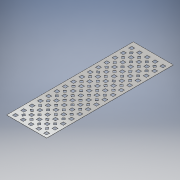
# Autodesk Inventor part: flat metal frame
Saved by Autodesk Inventor 2018 (Build 220112000, 112)
## iProperties
Created: 2018-10-16
Part Number: flat metal frame
Material: Generic
Document SubType Name: Modeling
Designer: USER
Density: 1 g/cm^3
Appearance: Machined - Aluminum
Author: USER
Autodesk Inventor part; units mm, degrees
ref_plane "YZ Plane" through (0, 0, 0) normal (1, 0, 0) x (0, 1, 0)
ref_plane "XZ Plane" through (0, 0, 0) normal (0, 1, 0) x (-1, 0, 0)
ref_plane "XY Plane" through (0, 0, 0) normal (0, 0, 1) x (1, 0, 0)
sketch "Sketch1" plane through (0, 0, 0) normal (0, 1, 0) x (-1, 0, 0)
  line L0 (0, 0) -> (59.9948, 0)
  line L1 (59.9948, 0) -> (59.9948, -189.992)
  line L2 (59.9948, -189.992) -> (0, -189.992)
  line L3 (0, -189.992) -> (0, 0)
  dimension "d0" = 59.9948
  dimension "d1" = 189.992
  constraints: 8 end point, 2 parallel, 1 horizontal, 1 perpendicular
  measures "d0" distance of L1.end L2.end
  measures "d1" distance of L0.end L1.end
extrude "Extrusion1" add sketch "Sketch1" against normal blind 0.254
sketch "Sketch2" plane through (0, 0, 0) normal (0, 1, 0) x (1, 0, 0)
  line L0 (-4.0386, 4.0386) -> (-8.6106, 4.0386)
  line L1 (-8.6106, 4.0386) -> (-8.6106, 8.6106)
  line L2 (-8.6106, 8.6106) -> (-4.0386, 8.6106)
  line L3 (-4.0386, 8.6106) -> (-4.0386, 4.0386)
  line L4 (-15.7226, 4.0386) -> (-20.2946, 4.0386)
  line L5 (-20.2946, 4.0386) -> (-20.2946, 8.6106)
  line L6 (-20.2946, 8.6106) -> (-15.7226, 8.6106)
  line L7 (-15.7226, 8.6106) -> (-15.7226, 4.0386)
  line L8 (-27.4066, 4.0386) -> (-31.9786, 4.0386)
  line L9 (-31.9786, 4.0386) -> (-31.9786, 8.6106)
  line L10 (-31.9786, 8.6106) -> (-27.4066, 8.6106)
  line L11 (-27.4066, 8.6106) -> (-27.4066, 4.0386)
  line L12 (-39.0906, 4.0386) -> (-43.6626, 4.0386)
  line L13 (-43.6626, 4.0386) -> (-43.6626, 8.6106)
  line L14 (-43.6626, 8.6106) -> (-39.0906, 8.6106)
  line L15 (-39.0906, 8.6106) -> (-39.0906, 4.0386)
  line L16 (-50.7746, 4.0386) -> (-55.3466, 4.0386)
  line L17 (-55.3466, 4.0386) -> (-55.3466, 8.6106)
  line L18 (-55.3466, 8.6106) -> (-50.7746, 8.6106)
  line L19 (-50.7746, 8.6106) -> (-50.7746, 4.0386)
  line L20 (-39.0906, 21.0566) -> (-39.0906, 16.4846)
  line L21 (-39.0906, 16.4846) -> (-43.6626, 16.4846)
  line L22 (-43.6626, 21.0566) -> (-39.0906, 21.0566)
  line L23 (-43.6626, 16.4846) -> (-43.6626, 21.0566)
  line L24 (-50.7746, 21.0566) -> (-50.7746, 16.4846)
  line L25 (-55.3466, 21.0566) -> (-50.7746, 21.0566)
  line L26 (-4.0386, 16.4846) -> (-8.6106, 16.4846)
  line L27 (-8.6106, 16.4846) -> (-8.6106, 21.0566)
  line L28 (-8.6106, 21.0566) -> (-4.0386, 21.0566)
  line L29 (-31.9786, 16.4846) -> (-31.9786, 21.0566)
  line L30 (-27.4066, 16.4846) -> (-31.9786, 16.4846)
  line L31 (-27.4066, 21.0566) -> (-27.4066, 16.4846)
  line L32 (-20.2946, 16.4846) -> (-20.2946, 21.0566)
  line L33 (-15.7226, 16.4846) -> (-20.2946, 16.4846)
  line L34 (-20.2946, 21.0566) -> (-15.7226, 21.0566)
  line L35 (-15.7226, 21.0566) -> (-15.7226, 16.4846)
  line L36 (-4.0386, 21.0566) -> (-4.0386, 16.4846)
  line L37 (-31.9786, 21.0566) -> (-27.4066, 21.0566)
  line L38 (-55.3466, 16.4846) -> (-55.3466, 21.0566)
  line L39 (-50.7746, 16.4846) -> (-55.3466, 16.4846)
  line L40 (-39.0906, 33.5026) -> (-39.0906, 28.9306)
  line L41 (-39.0906, 28.9306) -> (-43.6626, 28.9306)
  line L42 (-43.6626, 33.5026) -> (-39.0906, 33.5026)
  line L43 (-43.6626, 28.9306) -> (-43.6626, 33.5026)
  line L44 (-50.7746, 33.5026) -> (-50.7746, 28.9306)
  line L45 (-55.3466, 33.5026) -> (-50.7746, 33.5026)
  line L46 (-4.0386, 28.9306) -> (-8.6106, 28.9306)
  line L47 (-8.6106, 28.9306) -> (-8.6106, 33.5026)
  line L48 (-8.6106, 33.5026) -> (-4.0386, 33.5026)
  line L49 (-31.9786, 28.9306) -> (-31.9786, 33.5026)
  line L50 (-27.4066, 28.9306) -> (-31.9786, 28.9306)
  line L51 (-27.4066, 33.5026) -> (-27.4066, 28.9306)
  line L52 (-20.2946, 28.9306) -> (-20.2946, 33.5026)
  line L53 (-15.7226, 28.9306) -> (-20.2946, 28.9306)
  line L54 (-20.2946, 33.5026) -> (-15.7226, 33.5026)
  line L55 (-15.7226, 33.5026) -> (-15.7226, 28.9306)
  line L56 (-4.0386, 33.5026) -> (-4.0386, 28.9306)
  line L57 (-31.9786, 33.5026) -> (-27.4066, 33.5026)
  line L58 (-55.3466, 28.9306) -> (-55.3466, 33.5026)
  line L59 (-50.7746, 28.9306) -> (-55.3466, 28.9306)
  line L60 (-39.0906, 45.9486) -> (-39.0906, 41.3766)
  line L61 (-39.0906, 41.3766) -> (-43.6626, 41.3766)
  line L62 (-43.6626, 45.9486) -> (-39.0906, 45.9486)
  line L63 (-43.6626, 41.3766) -> (-43.6626, 45.9486)
  line L64 (-50.7746, 45.9486) -> (-50.7746, 41.3766)
  line L65 (-55.3466, 45.9486) -> (-50.7746, 45.9486)
  line L66 (-4.0386, 41.3766) -> (-8.6106, 41.3766)
  line L67 (-8.6106, 41.3766) -> (-8.6106, 45.9486)
  line L68 (-8.6106, 45.9486) -> (-4.0386, 45.9486)
  line L69 (-31.9786, 41.3766) -> (-31.9786, 45.9486)
  line L70 (-27.4066, 41.3766) -> (-31.9786, 41.3766)
  line L71 (-27.4066, 45.9486) -> (-27.4066, 41.3766)
  line L72 (-20.2946, 41.3766) -> (-20.2946, 45.9486)
  line L73 (-15.7226, 41.3766) -> (-20.2946, 41.3766)
  line L74 (-20.2946, 45.9486) -> (-15.7226, 45.9486)
  line L75 (-15.7226, 45.9486) -> (-15.7226, 41.3766)
  line L76 (-4.0386, 45.9486) -> (-4.0386, 41.3766)
  line L77 (-31.9786, 45.9486) -> (-27.4066, 45.9486)
  line L78 (-55.3466, 41.3766) -> (-55.3466, 45.9486)
  line L79 (-50.7746, 41.3766) -> (-55.3466, 41.3766)
  line L80 (-39.0906, 58.3946) -> (-39.0906, 53.8226)
  line L81 (-39.0906, 53.8226) -> (-43.6626, 53.8226)
  line L82 (-43.6626, 58.3946) -> (-39.0906, 58.3946)
  line L83 (-43.6626, 53.8226) -> (-43.6626, 58.3946)
  line L84 (-50.7746, 58.3946) -> (-50.7746, 53.8226)
  line L85 (-55.3466, 58.3946) -> (-50.7746, 58.3946)
  line L86 (-4.0386, 53.8226) -> (-8.6106, 53.8226)
  line L87 (-8.6106, 53.8226) -> (-8.6106, 58.3946)
  line L88 (-8.6106, 58.3946) -> (-4.0386, 58.3946)
  line L89 (-31.9786, 53.8226) -> (-31.9786, 58.3946)
  line L90 (-27.4066, 53.8226) -> (-31.9786, 53.8226)
  line L91 (-27.4066, 58.3946) -> (-27.4066, 53.8226)
  line L92 (-20.2946, 53.8226) -> (-20.2946, 58.3946)
  line L93 (-15.7226, 53.8226) -> (-20.2946, 53.8226)
  line L94 (-20.2946, 58.3946) -> (-15.7226, 58.3946)
  line L95 (-15.7226, 58.3946) -> (-15.7226, 53.8226)
  line L96 (-4.0386, 58.3946) -> (-4.0386, 53.8226)
  line L97 (-31.9786, 58.3946) -> (-27.4066, 58.3946)
  line L98 (-55.3466, 53.8226) -> (-55.3466, 58.3946)
  line L99 (-50.7746, 53.8226) -> (-55.3466, 53.8226)
  line L100 (-39.0906, 70.8406) -> (-39.0906, 66.2686)
  line L101 (-39.0906, 66.2686) -> (-43.6626, 66.2686)
  line L102 (-43.6626, 70.8406) -> (-39.0906, 70.8406)
  line L103 (-43.6626, 66.2686) -> (-43.6626, 70.8406)
  line L104 (-50.7746, 70.8406) -> (-50.7746, 66.2686)
  line L105 (-55.3466, 70.8406) -> (-50.7746, 70.8406)
  line L106 (-4.0386, 66.2686) -> (-8.6106, 66.2686)
  line L107 (-8.6106, 66.2686) -> (-8.6106, 70.8406)
  line L108 (-8.6106, 70.8406) -> (-4.0386, 70.8406)
  line L109 (-31.9786, 66.2686) -> (-31.9786, 70.8406)
  line L110 (-27.4066, 66.2686) -> (-31.9786, 66.2686)
  line L111 (-27.4066, 70.8406) -> (-27.4066, 66.2686)
  line L112 (-20.2946, 66.2686) -> (-20.2946, 70.8406)
  line L113 (-15.7226, 66.2686) -> (-20.2946, 66.2686)
  line L114 (-20.2946, 70.8406) -> (-15.7226, 70.8406)
  line L115 (-15.7226, 70.8406) -> (-15.7226, 66.2686)
  line L116 (-4.0386, 70.8406) -> (-4.0386, 66.2686)
  line L117 (-31.9786, 70.8406) -> (-27.4066, 70.8406)
  line L118 (-55.3466, 66.2686) -> (-55.3466, 70.8406)
  line L119 (-50.7746, 66.2686) -> (-55.3466, 66.2686)
  line L120 (-39.0906, 83.2866) -> (-39.0906, 78.7146)
  line L121 (-39.0906, 78.7146) -> (-43.6626, 78.7146)
  line L122 (-43.6626, 83.2866) -> (-39.0906, 83.2866)
  line L123 (-43.6626, 78.7146) -> (-43.6626, 83.2866)
  line L124 (-50.7746, 83.2866) -> (-50.7746, 78.7146)
  line L125 (-55.3466, 83.2866) -> (-50.7746, 83.2866)
  line L126 (-4.0386, 78.7146) -> (-8.6106, 78.7146)
  line L127 (-8.6106, 78.7146) -> (-8.6106, 83.2866)
  line L128 (-8.6106, 83.2866) -> (-4.0386, 83.2866)
  line L129 (-31.9786, 78.7146) -> (-31.9786, 83.2866)
  line L130 (-27.4066, 78.7146) -> (-31.9786, 78.7146)
  line L131 (-27.4066, 83.2866) -> (-27.4066, 78.7146)
  line L132 (-20.2946, 78.7146) -> (-20.2946, 83.2866)
  line L133 (-15.7226, 78.7146) -> (-20.2946, 78.7146)
  line L134 (-20.2946, 83.2866) -> (-15.7226, 83.2866)
  line L135 (-15.7226, 83.2866) -> (-15.7226, 78.7146)
  line L136 (-4.0386, 83.2866) -> (-4.0386, 78.7146)
  line L137 (-31.9786, 83.2866) -> (-27.4066, 83.2866)
  line L138 (-55.3466, 78.7146) -> (-55.3466, 83.2866)
  line L139 (-50.7746, 78.7146) -> (-55.3466, 78.7146)
  line L140 (-39.0906, 95.7326) -> (-39.0906, 91.1606)
  line L141 (-39.0906, 91.1606) -> (-43.6626, 91.1606)
  line L142 (-43.6626, 95.7326) -> (-39.0906, 95.7326)
  line L143 (-43.6626, 91.1606) -> (-43.6626, 95.7326)
  line L144 (-50.7746, 95.7326) -> (-50.7746, 91.1606)
  line L145 (-55.3466, 95.7326) -> (-50.7746, 95.7326)
  line L146 (-4.0386, 91.1606) -> (-8.6106, 91.1606)
  line L147 (-8.6106, 91.1606) -> (-8.6106, 95.7326)
  line L148 (-8.6106, 95.7326) -> (-4.0386, 95.7326)
  line L149 (-31.9786, 91.1606) -> (-31.9786, 95.7326)
  line L150 (-27.4066, 91.1606) -> (-31.9786, 91.1606)
  line L151 (-27.4066, 95.7326) -> (-27.4066, 91.1606)
  line L152 (-20.2946, 91.1606) -> (-20.2946, 95.7326)
  line L153 (-15.7226, 91.1606) -> (-20.2946, 91.1606)
  line L154 (-20.2946, 95.7326) -> (-15.7226, 95.7326)
  line L155 (-15.7226, 95.7326) -> (-15.7226, 91.1606)
  line L156 (-4.0386, 95.7326) -> (-4.0386, 91.1606)
  line L157 (-31.9786, 95.7326) -> (-27.4066, 95.7326)
  line L158 (-55.3466, 91.1606) -> (-55.3466, 95.7326)
  line L159 (-50.7746, 91.1606) -> (-55.3466, 91.1606)
  line L160 (-39.0906, 108.1786) -> (-39.0906, 103.6066)
  line L161 (-39.0906, 103.6066) -> (-43.6626, 103.6066)
  line L162 (-43.6626, 108.1786) -> (-39.0906, 108.1786)
  line L163 (-43.6626, 103.6066) -> (-43.6626, 108.1786)
  line L164 (-50.7746, 108.1786) -> (-50.7746, 103.6066)
  line L165 (-55.3466, 108.1786) -> (-50.7746, 108.1786)
  line L166 (-4.0386, 103.6066) -> (-8.6106, 103.6066)
  line L167 (-8.6106, 103.6066) -> (-8.6106, 108.1786)
  line L168 (-8.6106, 108.1786) -> (-4.0386, 108.1786)
  line L169 (-31.9786, 103.6066) -> (-31.9786, 108.1786)
  line L170 (-27.4066, 103.6066) -> (-31.9786, 103.6066)
  line L171 (-27.4066, 108.1786) -> (-27.4066, 103.6066)
  line L172 (-20.2946, 103.6066) -> (-20.2946, 108.1786)
  line L173 (-15.7226, 103.6066) -> (-20.2946, 103.6066)
  line L174 (-20.2946, 108.1786) -> (-15.7226, 108.1786)
  line L175 (-15.7226, 108.1786) -> (-15.7226, 103.6066)
  line L176 (-4.0386, 108.1786) -> (-4.0386, 103.6066)
  line L177 (-31.9786, 108.1786) -> (-27.4066, 108.1786)
  line L178 (-55.3466, 103.6066) -> (-55.3466, 108.1786)
  line L179 (-50.7746, 103.6066) -> (-55.3466, 103.6066)
  line L180 (-39.0906, 120.6246) -> (-39.0906, 116.0526)
  line L181 (-39.0906, 116.0526) -> (-43.6626, 116.0526)
  line L182 (-43.6626, 120.6246) -> (-39.0906, 120.6246)
  line L183 (-43.6626, 116.0526) -> (-43.6626, 120.6246)
  line L184 (-50.7746, 120.6246) -> (-50.7746, 116.0526)
  line L185 (-55.3466, 120.6246) -> (-50.7746, 120.6246)
  line L186 (-4.0386, 116.0526) -> (-8.6106, 116.0526)
  line L187 (-8.6106, 116.0526) -> (-8.6106, 120.6246)
  line L188 (-8.6106, 120.6246) -> (-4.0386, 120.6246)
  line L189 (-31.9786, 116.0526) -> (-31.9786, 120.6246)
  line L190 (-27.4066, 116.0526) -> (-31.9786, 116.0526)
  line L191 (-27.4066, 120.6246) -> (-27.4066, 116.0526)
  line L192 (-20.2946, 116.0526) -> (-20.2946, 120.6246)
  line L193 (-15.7226, 116.0526) -> (-20.2946, 116.0526)
  line L194 (-20.2946, 120.6246) -> (-15.7226, 120.6246)
  line L195 (-15.7226, 120.6246) -> (-15.7226, 116.0526)
  line L196 (-4.0386, 120.6246) -> (-4.0386, 116.0526)
  line L197 (-31.9786, 120.6246) -> (-27.4066, 120.6246)
  line L198 (-55.3466, 116.0526) -> (-55.3466, 120.6246)
  line L199 (-50.7746, 116.0526) -> (-55.3466, 116.0526)
  line L200 (-39.0906, 133.0706) -> (-39.0906, 128.4986)
  line L201 (-39.0906, 128.4986) -> (-43.6626, 128.4986)
  line L202 (-43.6626, 133.0706) -> (-39.0906, 133.0706)
  line L203 (-43.6626, 128.4986) -> (-43.6626, 133.0706)
  line L204 (-50.7746, 133.0706) -> (-50.7746, 128.4986)
  line L205 (-55.3466, 133.0706) -> (-50.7746, 133.0706)
  line L206 (-4.0386, 128.4986) -> (-8.6106, 128.4986)
  line L207 (-8.6106, 128.4986) -> (-8.6106, 133.0706)
  line L208 (-8.6106, 133.0706) -> (-4.0386, 133.0706)
  line L209 (-31.9786, 128.4986) -> (-31.9786, 133.0706)
  line L210 (-27.4066, 128.4986) -> (-31.9786, 128.4986)
  line L211 (-27.4066, 133.0706) -> (-27.4066, 128.4986)
  line L212 (-20.2946, 128.4986) -> (-20.2946, 133.0706)
  line L213 (-15.7226, 128.4986) -> (-20.2946, 128.4986)
  line L214 (-20.2946, 133.0706) -> (-15.7226, 133.0706)
  line L215 (-15.7226, 133.0706) -> (-15.7226, 128.4986)
  line L216 (-4.0386, 133.0706) -> (-4.0386, 128.4986)
  line L217 (-31.9786, 133.0706) -> (-27.4066, 133.0706)
  line L218 (-55.3466, 128.4986) -> (-55.3466, 133.0706)
  line L219 (-50.7746, 128.4986) -> (-55.3466, 128.4986)
  line L220 (-39.0906, 145.5166) -> (-39.0906, 140.9446)
  line L221 (-39.0906, 140.9446) -> (-43.6626, 140.9446)
  line L222 (-43.6626, 145.5166) -> (-39.0906, 145.5166)
  line L223 (-43.6626, 140.9446) -> (-43.6626, 145.5166)
  line L224 (-50.7746, 145.5166) -> (-50.7746, 140.9446)
  line L225 (-55.3466, 145.5166) -> (-50.7746, 145.5166)
  line L226 (-4.0386, 140.9446) -> (-8.6106, 140.9446)
  line L227 (-8.6106, 140.9446) -> (-8.6106, 145.5166)
  line L228 (-8.6106, 145.5166) -> (-4.0386, 145.5166)
  line L229 (-31.9786, 140.9446) -> (-31.9786, 145.5166)
  line L230 (-27.4066, 140.9446) -> (-31.9786, 140.9446)
  line L231 (-27.4066, 145.5166) -> (-27.4066, 140.9446)
  line L232 (-20.2946, 140.9446) -> (-20.2946, 145.5166)
  line L233 (-15.7226, 140.9446) -> (-20.2946, 140.9446)
  line L234 (-20.2946, 145.5166) -> (-15.7226, 145.5166)
  line L235 (-15.7226, 145.5166) -> (-15.7226, 140.9446)
  line L236 (-4.0386, 145.5166) -> (-4.0386, 140.9446)
  line L237 (-31.9786, 145.5166) -> (-27.4066, 145.5166)
  line L238 (-55.3466, 140.9446) -> (-55.3466, 145.5166)
  line L239 (-50.7746, 140.9446) -> (-55.3466, 140.9446)
  line L240 (-39.0906, 157.9626) -> (-39.0906, 153.3906)
  line L241 (-39.0906, 153.3906) -> (-43.6626, 153.3906)
  line L242 (-43.6626, 157.9626) -> (-39.0906, 157.9626)
  line L243 (-43.6626, 153.3906) -> (-43.6626, 157.9626)
  line L244 (-50.7746, 157.9626) -> (-50.7746, 153.3906)
  line L245 (-55.3466, 157.9626) -> (-50.7746, 157.9626)
  line L246 (-4.0386, 153.3906) -> (-8.6106, 153.3906)
  line L247 (-8.6106, 153.3906) -> (-8.6106, 157.9626)
  line L248 (-8.6106, 157.9626) -> (-4.0386, 157.9626)
  line L249 (-31.9786, 153.3906) -> (-31.9786, 157.9626)
  line L250 (-27.4066, 153.3906) -> (-31.9786, 153.3906)
  line L251 (-27.4066, 157.9626) -> (-27.4066, 153.3906)
  line L252 (-20.2946, 153.3906) -> (-20.2946, 157.9626)
  line L253 (-15.7226, 153.3906) -> (-20.2946, 153.3906)
  line L254 (-20.2946, 157.9626) -> (-15.7226, 157.9626)
  line L255 (-15.7226, 157.9626) -> (-15.7226, 153.3906)
  line L256 (-4.0386, 157.9626) -> (-4.0386, 153.3906)
  line L257 (-31.9786, 157.9626) -> (-27.4066, 157.9626)
  line L258 (-55.3466, 153.3906) -> (-55.3466, 157.9626)
  line L259 (-50.7746, 153.3906) -> (-55.3466, 153.3906)
  line L260 (-39.0906, 170.4086) -> (-39.0906, 165.8366)
  line L261 (-39.0906, 165.8366) -> (-43.6626, 165.8366)
  line L262 (-43.6626, 170.4086) -> (-39.0906, 170.4086)
  line L263 (-43.6626, 165.8366) -> (-43.6626, 170.4086)
  line L264 (-50.7746, 170.4086) -> (-50.7746, 165.8366)
  line L265 (-55.3466, 170.4086) -> (-50.7746, 170.4086)
  line L266 (-4.0386, 165.8366) -> (-8.6106, 165.8366)
  line L267 (-8.6106, 165.8366) -> (-8.6106, 170.4086)
  line L268 (-8.6106, 170.4086) -> (-4.0386, 170.4086)
  line L269 (-31.9786, 165.8366) -> (-31.9786, 170.4086)
  line L270 (-27.4066, 165.8366) -> (-31.9786, 165.8366)
  line L271 (-27.4066, 170.4086) -> (-27.4066, 165.8366)
  line L272 (-20.2946, 165.8366) -> (-20.2946, 170.4086)
  line L273 (-15.7226, 165.8366) -> (-20.2946, 165.8366)
  line L274 (-20.2946, 170.4086) -> (-15.7226, 170.4086)
  line L275 (-15.7226, 170.4086) -> (-15.7226, 165.8366)
  line L276 (-4.0386, 170.4086) -> (-4.0386, 165.8366)
  line L277 (-31.9786, 170.4086) -> (-27.4066, 170.4086)
  line L278 (-55.3466, 165.8366) -> (-55.3466, 170.4086)
  line L279 (-50.7746, 165.8366) -> (-55.3466, 165.8366)
  line L280 (-39.0906, 182.8546) -> (-39.0906, 178.2826)
  line L281 (-39.0906, 178.2826) -> (-43.6626, 178.2826)
  line L282 (-43.6626, 182.8546) -> (-39.0906, 182.8546)
  line L283 (-43.6626, 178.2826) -> (-43.6626, 182.8546)
  line L284 (-50.7746, 182.8546) -> (-50.7746, 178.2826)
  line L285 (-55.3466, 182.8546) -> (-50.7746, 182.8546)
  line L286 (-4.0386, 178.2826) -> (-8.6106, 178.2826)
  line L287 (-8.6106, 178.2826) -> (-8.6106, 182.8546)
  line L288 (-8.6106, 182.8546) -> (-4.0386, 182.8546)
  line L289 (-31.9786, 178.2826) -> (-31.9786, 182.8546)
  line L290 (-27.4066, 178.2826) -> (-31.9786, 178.2826)
  line L291 (-27.4066, 182.8546) -> (-27.4066, 178.2826)
  line L292 (-20.2946, 178.2826) -> (-20.2946, 182.8546)
  line L293 (-15.7226, 178.2826) -> (-20.2946, 178.2826)
  line L294 (-20.2946, 182.8546) -> (-15.7226, 182.8546)
  line L295 (-15.7226, 182.8546) -> (-15.7226, 178.2826)
  line L296 (-4.0386, 182.8546) -> (-4.0386, 178.2826)
  line L297 (-31.9786, 182.8546) -> (-27.4066, 182.8546)
  line L298 (-55.3466, 178.2826) -> (-55.3466, 182.8546)
  line L299 (-50.7746, 178.2826) -> (-55.3466, 178.2826)
  line L300 (-9.6789, 12.6578) -> (-12.1161, 15.2472)
  line L301 (-12.1161, 15.2472) -> (-14.7055, 12.8099)
  line L302 (-14.7055, 12.8099) -> (-12.2682, 10.2205)
  line L303 (-12.2682, 10.2205) -> (-9.6789, 12.6578)
  line L304 (-9.6789, 12.6578) -> (-14.7055, 12.8099) construction
  line L305 (-12.1161, 15.2472) -> (-12.2682, 10.2205) construction
  line L306 (-26.3383, 12.6578) -> (-23.9011, 15.2472)
  line L307 (-23.9011, 15.2472) -> (-21.3117, 12.8099)
  line L308 (-21.3117, 12.8099) -> (-23.749, 10.2205)
  line L309 (-23.749, 10.2205) -> (-26.3383, 12.6578)
  line L310 (-38.0735, 12.8099) -> (-35.6362, 10.2205)
  line L311 (-35.4841, 15.2472) -> (-38.0735, 12.8099)
  line L312 (-33.0469, 12.6578) -> (-35.4841, 15.2472)
  line L313 (-35.6362, 10.2205) -> (-33.0469, 12.6578)
  line L314 (-47.117, 10.2205) -> (-49.7063, 12.6578)
  line L315 (-49.7063, 12.6578) -> (-47.2691, 15.2472)
  line L316 (-47.2691, 15.2472) -> (-44.6797, 12.8099)
  line L317 (-44.6797, 12.8099) -> (-47.117, 10.2205)
  line L318 (-9.6789, 24.8834) -> (-12.1161, 22.294)
  line L319 (-12.1161, 22.294) -> (-14.7055, 24.7313)
  line L320 (-14.7055, 24.7313) -> (-12.2682, 27.3207)
  line L321 (-12.2682, 27.3207) -> (-9.6789, 24.8834)
  line L322 (-21.3117, 24.7313) -> (-23.749, 27.3207)
  line L323 (-23.9011, 22.294) -> (-21.3117, 24.7313)
  line L324 (-26.3383, 24.8834) -> (-23.9011, 22.294)
  line L325 (-23.749, 27.3207) -> (-26.3383, 24.8834)
  line L326 (-35.6362, 27.3207) -> (-33.0469, 24.8834)
  line L327 (-33.0469, 24.8834) -> (-35.4841, 22.294)
  line L328 (-35.4841, 22.294) -> (-38.0735, 24.7313)
  line L329 (-38.0735, 24.7313) -> (-35.6362, 27.3207)
  line L330 (-44.6797, 24.7313) -> (-47.117, 27.3207)
  line L331 (-47.2691, 22.294) -> (-44.6797, 24.7313)
  line L332 (-49.7063, 24.8834) -> (-47.2691, 22.294)
  line L333 (-47.117, 27.3207) -> (-49.7063, 24.8834)
  line L334 (-44.6797, 37.7019) -> (-47.117, 35.1125)
  line L335 (-47.117, 35.1125) -> (-49.7063, 37.5498)
  line L336 (-49.7063, 37.5498) -> (-47.2691, 40.1392)
  line L337 (-47.2691, 40.1392) -> (-44.6797, 37.7019)
  line L338 (-38.0735, 37.7019) -> (-35.6362, 35.1125)
  line L339 (-35.4841, 40.1392) -> (-38.0735, 37.7019)
  line L340 (-33.0469, 37.5498) -> (-35.4841, 40.1392)
  line L341 (-35.6362, 35.1125) -> (-33.0469, 37.5498)
  line L342 (-23.749, 35.1125) -> (-26.3383, 37.5498)
  line L343 (-26.3383, 37.5498) -> (-23.9011, 40.1392)
  line L344 (-23.9011, 40.1392) -> (-21.3117, 37.7019)
  line L345 (-21.3117, 37.7019) -> (-23.749, 35.1125)
  line L346 (-14.7055, 37.7019) -> (-12.2682, 35.1125)
  line L347 (-12.1161, 40.1392) -> (-14.7055, 37.7019)
  line L348 (-9.6789, 37.5498) -> (-12.1161, 40.1392)
  line L349 (-12.2682, 35.1125) -> (-9.6789, 37.5498)
  line L350 (-9.6789, 74.6674) -> (-12.1161, 72.078)
  line L351 (-12.1161, 72.078) -> (-14.7055, 74.5153)
  line L352 (-14.7055, 74.5153) -> (-12.2682, 77.1047)
  line L353 (-12.2682, 77.1047) -> (-9.6789, 74.6674)
  line L354 (-9.6789, 74.6674) -> (-14.7055, 74.5153) construction
  line L355 (-12.1161, 72.078) -> (-12.2682, 77.1047) construction
  line L356 (-21.3117, 74.5153) -> (-23.749, 77.1047)
  line L357 (-23.9011, 72.078) -> (-21.3117, 74.5153)
  line L358 (-26.3383, 74.6674) -> (-23.9011, 72.078)
  line L359 (-23.749, 77.1047) -> (-26.3383, 74.6674)
  line L360 (-35.6362, 77.1047) -> (-33.0469, 74.6674)
  line L361 (-33.0469, 74.6674) -> (-35.4841, 72.078)
  line L362 (-35.4841, 72.078) -> (-38.0735, 74.5153)
  line L363 (-38.0735, 74.5153) -> (-35.6362, 77.1047)
  line L364 (-44.6797, 74.5153) -> (-47.117, 77.1047)
  line L365 (-47.2691, 72.078) -> (-44.6797, 74.5153)
  line L366 (-49.7063, 74.6674) -> (-47.2691, 72.078)
  line L367 (-47.117, 77.1047) -> (-49.7063, 74.6674)
  line L368 (-44.6797, 62.5939) -> (-47.117, 60.0045)
  line L369 (-47.117, 60.0045) -> (-49.7063, 62.4418)
  line L370 (-49.7063, 62.4418) -> (-47.2691, 65.0312)
  line L371 (-47.2691, 65.0312) -> (-44.6797, 62.5939)
  line L372 (-38.0735, 62.5939) -> (-35.6362, 60.0045)
  line L373 (-35.4841, 65.0312) -> (-38.0735, 62.5939)
  line L374 (-33.0469, 62.4418) -> (-35.4841, 65.0312)
  line L375 (-35.6362, 60.0045) -> (-33.0469, 62.4418)
  line L376 (-23.749, 60.0045) -> (-26.3383, 62.4418)
  line L377 (-26.3383, 62.4418) -> (-23.9011, 65.0312)
  line L378 (-23.9011, 65.0312) -> (-21.3117, 62.5939)
  line L379 (-21.3117, 62.5939) -> (-23.749, 60.0045)
  line L380 (-14.7055, 62.5939) -> (-12.2682, 60.0045)
  line L381 (-12.1161, 65.0312) -> (-14.7055, 62.5939)
  line L382 (-9.6789, 62.4418) -> (-12.1161, 65.0312)
  line L383 (-12.2682, 60.0045) -> (-9.6789, 62.4418)
  line L384 (-49.7063, 49.7754) -> (-47.2691, 47.186)
  line L385 (-47.117, 52.2127) -> (-49.7063, 49.7754)
  line L386 (-44.6797, 49.6233) -> (-47.117, 52.2127)
  line L387 (-47.2691, 47.186) -> (-44.6797, 49.6233)
  line L388 (-35.4841, 47.186) -> (-38.0735, 49.6233)
  line L389 (-38.0735, 49.6233) -> (-35.6362, 52.2127)
  line L390 (-35.6362, 52.2127) -> (-33.0469, 49.7754)
  line L391 (-33.0469, 49.7754) -> (-35.4841, 47.186)
  line L392 (-26.3383, 49.7754) -> (-23.9011, 47.186)
  line L393 (-23.749, 52.2127) -> (-26.3383, 49.7754)
  line L394 (-21.3117, 49.6233) -> (-23.749, 52.2127)
  line L395 (-23.9011, 47.186) -> (-21.3117, 49.6233)
  line L396 (-12.1161, 47.186) -> (-14.7055, 49.6233)
  line L397 (-14.7055, 49.6233) -> (-12.2682, 52.2127)
  line L398 (-12.2682, 52.2127) -> (-9.6789, 49.7754)
  line L399 (-9.6789, 49.7754) -> (-12.1161, 47.186)
  line L400 (-9.6789, 149.3434) -> (-12.1161, 146.754)
  line L401 (-12.1161, 146.754) -> (-14.7055, 149.1913)
  line L402 (-14.7055, 149.1913) -> (-12.2682, 151.7807)
  line L403 (-12.2682, 151.7807) -> (-9.6789, 149.3434)
  line L404 (-9.6789, 149.3434) -> (-14.7055, 149.1913) construction
  line L405 (-12.1161, 146.754) -> (-12.2682, 151.7807) construction
  line L406 (-21.3117, 149.1913) -> (-23.749, 151.7807)
  line L407 (-23.9011, 146.754) -> (-21.3117, 149.1913)
  line L408 (-26.3383, 149.3434) -> (-23.9011, 146.754)
  line L409 (-23.749, 151.7807) -> (-26.3383, 149.3434)
  line L410 (-35.6362, 151.7807) -> (-33.0469, 149.3434)
  line L411 (-33.0469, 149.3434) -> (-35.4841, 146.754)
  line L412 (-35.4841, 146.754) -> (-38.0735, 149.1913)
  line L413 (-38.0735, 149.1913) -> (-35.6362, 151.7807)
  line L414 (-44.6797, 149.1913) -> (-47.117, 151.7807)
  line L415 (-47.2691, 146.754) -> (-44.6797, 149.1913)
  line L416 (-49.7063, 149.3434) -> (-47.2691, 146.754)
  line L417 (-47.117, 151.7807) -> (-49.7063, 149.3434)
  line L418 (-44.6797, 137.2699) -> (-47.117, 134.6805)
  line L419 (-47.117, 134.6805) -> (-49.7063, 137.1178)
  line L420 (-49.7063, 137.1178) -> (-47.2691, 139.7072)
  line L421 (-47.2691, 139.7072) -> (-44.6797, 137.2699)
  line L422 (-38.0735, 137.2699) -> (-35.6362, 134.6805)
  line L423 (-35.4841, 139.7072) -> (-38.0735, 137.2699)
  line L424 (-33.0469, 137.1178) -> (-35.4841, 139.7072)
  line L425 (-35.6362, 134.6805) -> (-33.0469, 137.1178)
  line L426 (-23.749, 134.6805) -> (-26.3383, 137.1178)
  line L427 (-26.3383, 137.1178) -> (-23.9011, 139.7072)
  line L428 (-23.9011, 139.7072) -> (-21.3117, 137.2699)
  line L429 (-21.3117, 137.2699) -> (-23.749, 134.6805)
  line L430 (-14.7055, 137.2699) -> (-12.2682, 134.6805)
  line L431 (-12.1161, 139.7072) -> (-14.7055, 137.2699)
  line L432 (-9.6789, 137.1178) -> (-12.1161, 139.7072)
  line L433 (-12.2682, 134.6805) -> (-9.6789, 137.1178)
  line L434 (-49.7063, 124.4514) -> (-47.2691, 121.862)
  line L435 (-47.117, 126.8887) -> (-49.7063, 124.4514)
  line L436 (-44.6797, 124.2993) -> (-47.117, 126.8887)
  line L437 (-47.2691, 121.862) -> (-44.6797, 124.2993)
  line L438 (-35.4841, 121.862) -> (-38.0735, 124.2993)
  line L439 (-38.0735, 124.2993) -> (-35.6362, 126.8887)
  line L440 (-35.6362, 126.8887) -> (-33.0469, 124.4514)
  line L441 (-33.0469, 124.4514) -> (-35.4841, 121.862)
  line L442 (-26.3383, 124.4514) -> (-23.9011, 121.862)
  line L443 (-23.749, 126.8887) -> (-26.3383, 124.4514)
  line L444 (-21.3117, 124.2993) -> (-23.749, 126.8887)
  line L445 (-23.9011, 121.862) -> (-21.3117, 124.2993)
  line L446 (-12.1161, 121.862) -> (-14.7055, 124.2993)
  line L447 (-14.7055, 124.2993) -> (-12.2682, 126.8887)
  line L448 (-12.2682, 126.8887) -> (-9.6789, 124.4514)
  line L449 (-9.6789, 124.4514) -> (-12.1161, 121.862)
  line L450 (-47.117, 84.8965) -> (-49.7063, 87.3338)
  line L451 (-49.7063, 87.3338) -> (-47.2691, 89.9232)
  line L452 (-47.2691, 89.9232) -> (-44.6797, 87.4859)
  line L453 (-44.6797, 87.4859) -> (-47.117, 84.8965)
  line L454 (-49.7063, 99.5594) -> (-47.2691, 96.97)
  line L455 (-47.2691, 96.97) -> (-44.6797, 99.4073)
  line L456 (-44.6797, 99.4073) -> (-47.117, 101.9967)
  line L457 (-47.117, 101.9967) -> (-49.7063, 99.5594)
  line L458 (-47.2691, 114.8152) -> (-44.6797, 112.3779)
  line L459 (-49.7063, 112.2258) -> (-47.2691, 114.8152)
  line L460 (-47.117, 109.7885) -> (-49.7063, 112.2258)
  line L461 (-44.6797, 112.3779) -> (-47.117, 109.7885)
  line L462 (-35.4841, 114.8152) -> (-38.0735, 112.3779)
  line L463 (-33.0469, 112.2258) -> (-35.4841, 114.8152)
  line L464 (-35.6362, 109.7885) -> (-33.0469, 112.2258)
  line L465 (-38.0735, 112.3779) -> (-35.6362, 109.7885)
  line L466 (-38.0735, 99.4073) -> (-35.6362, 101.9967)
  line L467 (-35.6362, 101.9967) -> (-33.0469, 99.5594)
  line L468 (-33.0469, 99.5594) -> (-35.4841, 96.97)
  line L469 (-35.4841, 96.97) -> (-38.0735, 99.4073)
  line L470 (-35.4841, 89.9232) -> (-38.0735, 87.4859)
  line L471 (-33.0469, 87.3338) -> (-35.4841, 89.9232)
  line L472 (-38.0735, 87.4859) -> (-35.6362, 84.8965)
  line L473 (-35.6362, 84.8965) -> (-33.0469, 87.3338)
  line L474 (-21.3117, 87.4859) -> (-23.749, 84.8965)
  line L475 (-23.9011, 89.9232) -> (-21.3117, 87.4859)
  line L476 (-23.749, 84.8965) -> (-26.3383, 87.3338)
  line L477 (-26.3383, 87.3338) -> (-23.9011, 89.9232)
  line L478 (-23.9011, 96.97) -> (-21.3117, 99.4073)
  line L479 (-26.3383, 99.5594) -> (-23.9011, 96.97)
  line L480 (-21.3117, 99.4073) -> (-23.749, 101.9967)
  line L481 (-23.749, 101.9967) -> (-26.3383, 99.5594)
  line L482 (-21.3117, 112.3779) -> (-23.749, 109.7885)
  line L483 (-23.9011, 114.8152) -> (-21.3117, 112.3779)
  line L484 (-23.749, 109.7885) -> (-26.3383, 112.2258)
  line L485 (-26.3383, 112.2258) -> (-23.9011, 114.8152)
  line L486 (-14.7055, 112.3779) -> (-12.2682, 109.7885)
  line L487 (-12.1161, 114.8152) -> (-14.7055, 112.3779)
  line L488 (-9.6789, 112.2258) -> (-12.1161, 114.8152)
  line L489 (-12.2682, 109.7885) -> (-9.6789, 112.2258)
  line L490 (-12.1161, 96.97) -> (-14.7055, 99.4073)
  line L491 (-9.6789, 99.5594) -> (-12.1161, 96.97)
  line L492 (-12.2682, 101.9967) -> (-9.6789, 99.5594)
  line L493 (-14.7055, 99.4073) -> (-12.2682, 101.9967)
  line L494 (-12.1161, 89.9232) -> (-14.7055, 87.4859)
  line L495 (-14.7055, 87.4859) -> (-12.2682, 84.8965)
  line L496 (-12.1161, 89.9232) -> (-12.2682, 84.8965) construction
  line L497 (-9.6789, 87.3338) -> (-14.7055, 87.4859) construction
  line L498 (-9.6789, 87.3338) -> (-12.1161, 89.9232)
  line L499 (-12.2682, 84.8965) -> (-9.6789, 87.3338)
  line L500 (-55.3466, 155.6766) -> (-4.0386, 155.6766)
  line L501 (-44.6797, 162.1619) -> (-47.117, 159.5725)
  line L502 (-47.2691, 164.5992) -> (-44.6797, 162.1619)
  line L503 (-49.7063, 162.0098) -> (-47.2691, 164.5992)
  line L504 (-47.117, 159.5725) -> (-49.7063, 162.0098)
  line L505 (-44.6797, 174.0833) -> (-47.117, 176.6727)
  line L506 (-47.2691, 171.646) -> (-44.6797, 174.0833)
  line L507 (-49.7063, 174.2354) -> (-47.2691, 171.646)
  line L508 (-47.117, 176.6727) -> (-49.7063, 174.2354)
  line L509 (-38.0735, 162.1619) -> (-35.6362, 159.5725)
  line L510 (-35.4841, 164.5992) -> (-38.0735, 162.1619)
  line L511 (-33.0469, 162.0098) -> (-35.4841, 164.5992)
  line L512 (-35.6362, 159.5725) -> (-33.0469, 162.0098)
  line L513 (-38.0735, 174.0833) -> (-35.6362, 176.6727)
  line L514 (-35.4841, 171.646) -> (-38.0735, 174.0833)
  line L515 (-33.0469, 174.2354) -> (-35.4841, 171.646)
  line L516 (-35.6362, 176.6727) -> (-33.0469, 174.2354)
  line L517 (-23.9011, 171.646) -> (-21.3117, 174.0833)
  line L518 (-26.3383, 174.2354) -> (-23.9011, 171.646)
  line L519 (-23.749, 176.6727) -> (-26.3383, 174.2354)
  line L520 (-21.3117, 174.0833) -> (-23.749, 176.6727)
  line L521 (-26.3383, 162.0098) -> (-23.9011, 164.5992)
  line L522 (-23.749, 159.5725) -> (-26.3383, 162.0098)
  line L523 (-21.3117, 162.1619) -> (-23.749, 159.5725)
  line L524 (-23.9011, 164.5992) -> (-21.3117, 162.1619)
  line L525 (-12.2682, 159.5725) -> (-9.6789, 162.0098)
  line L526 (-14.7055, 162.1619) -> (-12.2682, 159.5725)
  line L527 (-12.1161, 164.5992) -> (-12.2682, 159.5725) construction
  line L528 (-9.6789, 162.0098) -> (-12.1161, 164.5992)
  line L529 (-9.6789, 162.0098) -> (-14.7055, 162.1619) construction
  line L530 (-12.1161, 164.5992) -> (-14.7055, 162.1619)
  line L531 (-12.1161, 171.646) -> (-14.7055, 174.0833)
  line L532 (-9.6789, 174.2354) -> (-12.1161, 171.646)
  line L533 (-14.7055, 174.0833) -> (-12.2682, 176.6727)
  line L534 (-12.2682, 176.6727) -> (-9.6789, 174.2354)
  point P0 (0, 0)
  point P1 (-12.1922, 12.7339)
  point P2 (-55.3466, 18.7706)
  point P3 (-55.3466, 31.2166)
  point P4 (-12.1922, 74.5913)
  point P5 (-12.1922, 149.2673)
  point P6 (-12.1922, 87.4099)
  point P7 (-12.1922, 162.0859)
  dimension "d4" = 4.572
  dimension "d5" = 4.572
  dimension "d11" = 11.684
  dimension "d18" = 12.446
  dimension "d20" = 3.556
  dimension "d21" = 3.556
  constraints: 1070 end point, 33 symmetric about line, 14 midpoint, 4 parallel, 2 collinear, 2 horizontal, 2 perpendicular, 1 vertical, 590 other
  measures "d4" distance of L1.end L2.end
  measures "d5" distance of L0.end L1.end
  measures "d11" distance of L0.start L4.start
  measures "d18" distance of L12.start L20.end
  measures "d20" distance of L300.start L300.end
  measures "d21" distance of L301.end L300.end
extrude "Extrusion2" cut sketch "Sketch2" against normal through all
body "Solid1"
